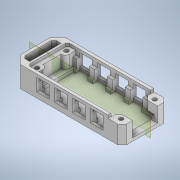
# Autodesk Inventor part: Case_main
Saved by Autodesk Inventor 2020 (Build 240168000, 168)
## iProperties
Created: 2022-03-19
Part Number: Case_main
Material: Типовые
Document SubType Name: Modeling
Designer: NoName
Density: 1 g/cm^3
Appearance: По умолчанию
Author: NoName
Autodesk Inventor part; units mm, degrees
ref_plane "YZ Plane" through (0, 0, 0) normal (1, 0, 0) x (0, 1, 0)
ref_plane "XZ Plane" through (0, 0, 0) normal (0, 1, 0) x (-1, 0, 0)
sketch "Эскиз1" plane through (0, 0, 0) normal (0, 1, 0) x (-1, 0, 0)
  line L0 (0, 0) -> (0, -19)
  line L1 (0, -19) -> (40.8, -19)
  line L2 (40.8, -19) -> (40.8, -15.85)
  arc A0 (42.8, -13.85) -> (40.8, -15.85) centre (42.8, -15.85) ccw
  line L3 (42.8, -15.85) -> (42.8, -13.85) construction
  line L4 (42.8, -15.85) -> (40.8, -15.85) construction
  line L5 (42.8, -13.85) -> (42.8, -5.15)
  line L6 (42.8, -9.5) -> (0, -9.5)
  line L7 (0, 0) -> (40.8, 0)
  line L8 (40.8, 0) -> (40.8, -3.15)
  arc A1 (40.8, -3.15) -> (42.8, -5.15) centre (42.8, -3.15) ccw
  line L9 (42.8, -3.15) -> (42.8, -5.15) construction
  line L10 (42.8, -3.15) -> (40.8, -3.15) construction
  line L11 (46.8, -20.4) -> (0.4, -20.4)
  line L12 (46.8, 1.4) -> (0.4, 1.4)
  line L13 (50.8, -16.4) -> (50.8, -2.6)
  line L14 (45.8, -17) -> (45.8, -2)
  line L15 (49.3, -15.7787) -> (49.3, -3.2213)
  line L16 (5.1, -19) -> (5.1, -17.6)
  line L17 (5.1, -17.6) -> (0, -17.6)
  line L18 (5.1, 0) -> (5.1, -1.4)
  line L19 (5.1, -1.4) -> (0, -1.4)
  line L20 (0.4, -20.4) -> (-1.6, -18.4)
  line L21 (-1.6, -18.4) -> (-1.6, -0.6)
  line L22 (-1.6, -0.6) -> (0.4, 1.4)
  line L23 (46.8, 1.4) -> (50.8, -2.6)
  line L24 (50.8, -16.4) -> (46.8, -20.4)
  line L25 (49.3, -15.7787) -> (48.0787, -17)
  line L26 (48.0787, -17) -> (45.8, -17)
  line L27 (49.3, -3.2213) -> (48.0787, -2)
  line L28 (48.0787, -2) -> (45.8, -2)
  point P0 (5.1, 0)
  point P1 (0, -1.4)
  point P2 (45.8, -9.5)
  point P3 (49.3, -9.5)
  point P4 (50.8, -9.5)
  dimension "d1" = 42.8
  dimension "d3" = 2
  dimension "d4" = 12.7
  dimension "d8" = 19
  dimension "d12" = 3.5
  dimension "d32" = 21.8
  dimension "d34" = 5.1
  dimension "d35" = 16.2
  dimension "d41" = 135
  dimension "d42" = 1.6
  dimension "d43" = 2
  dimension "d65" = 8
  dimension "d66" = 1.5
  dimension "d67" = 15
  dimension "d68" = 1.5
  dimension "d69" = 4
  constraints: 59 end point, 13 symmetric about line, 7 vertical, 6 perpendicular, 5 midpoint, 4 point on circle, 3 horizontal alignment, 2 centre point, 2 point on line, 1 horizontal, 1 parallel, 1 tangent, 1 other
  measures "d1" distance between parallel lines of L0 L5
  measures "d3" distance between parallel lines of L5 L8
  measures "d4" distance of L9.start L3.start
  measures "d8" distance between parallel lines of L7 L1
  measures "d12" distance between parallel lines of L15 L14
  measures "d32" distance between parallel lines of L12 L11
  measures "d34" distance between parallel lines of L0 L16
  measures "d35" distance between parallel lines of L19 L17
  measures "d41" angle of L12 L22
  measures "d42" distance between parallel lines of L0 L21
  measures "d43" horizontal distance of L21.end L12.end
  measures "d65" distance between parallel lines of L5 L13
  measures "d66" distance between parallel lines of L13 L15
  measures "d67" distance between parallel lines of L28 L26
  measures "d68" distance between parallel lines of L24 L25
  measures "d69" distance from line of L5 L11.start
extrude "Выдавливание1" add sketch "Эскиз1" along normal blind 6 contours L7 L18 L19 L0 | L17 L16 L1 L0 | L11 L20 L21 L22 L12 L23 L13 L24
sketch "Эскиз2" plane through (0, 0, 0) normal (0, -1, 0) x (1, 0, 0)
  line L0 (-0.4, -20.4) -> (-46.8, -20.4) projected
  line L1 (-46.8, 1.4) -> (-0.4, 1.4) projected
  line L2 (-50.8, -16.4) -> (-50.8, -2.6) projected
  line L3 (-42.8, -5.15) -> (-42.8, -13.85) projected
  arc A0 (-42.8, -5.15) -> (-40.8, -3.15) centre (-42.8, -3.15) ccw projected
  line L4 (-40.8, 0) -> (-40.8, -3.15) projected
  line L5 (-5.1, 0) -> (-40.8, 0) projected
  line L6 (0, -17.6) -> (0, -1.4) projected
  line L7 (-40.8, -19) -> (-5.1, -19) projected
  line L8 (-40.8, -15.85) -> (-40.8, -19) projected
  arc A1 (-40.8, -15.85) -> (-42.8, -13.85) centre (-42.8, -15.85) ccw projected
  line L9 (-40.8, -15.85) -> (-40.8, -19) projected
  line L10 (-40.8, -19) -> (-5.1, -19) projected
  line L11 (-39.8, -16.8) -> (-1.5, -16.8)
  line L12 (-1.5, -16.8) -> (-1.5, -2.2)
  line L13 (-1.5, -2.2) -> (-39.8, -2.2)
  line L14 (-39.8, -2.2) -> (-39.8, -16.8)
  line L15 (-5.1, -1.4) -> (-5.1, 0) projected
  line L16 (0, -1.4) -> (-5.1, -1.4) projected
  line L17 (-5.1, -17.6) -> (0, -17.6) projected
  line L18 (-5.1, -19) -> (-5.1, -17.6) projected
  line L19 (1.6, -18.4) -> (-0.4, -20.4) projected
  line L20 (1.6, -0.6) -> (1.6, -18.4) projected
  line L21 (-0.4, 1.4) -> (1.6, -0.6) projected
  line L22 (-50.8, -2.6) -> (-46.8, 1.4) projected
  line L23 (-46.8, -20.4) -> (-50.8, -16.4) projected
  line L24 (-49.3, -3.2213) -> (-49.3, -15.7787) projected
  line L25 (-48.0787, -2) -> (-49.3, -3.2213) projected
  line L26 (-45.8, -2) -> (-48.0787, -2) projected
  line L27 (-45.8, -17) -> (-45.8, -2) projected
  line L28 (-48.0787, -17) -> (-45.8, -17) projected
  line L29 (-49.3, -15.7787) -> (-48.0787, -17) projected
  point P0 (0, -18.2)
  point P1 (-42.8, -9.5)
  point P2 (-39.8, -9.5)
  dimension "d17" = 1.5
  dimension "d18" = 3
  dimension "d33" = 14.6
  constraints: 8 end point, 2 midpoint, 2 parallel, 1 horizontal, 1 horizontal alignment, 1 perpendicular, 1 other
  measures "d17" distance between parallel lines of L6 L12
  measures "d18" distance between parallel lines of L3 L14
  measures "d33" distance between parallel lines of L13 L11
extrude "Выдавливание2" add sketch "Эскиз2" along normal blind 1.6 contours L0 L23 L2 L22 L1 L21 L20 L19 | A0 L4 L5 L15 L16 L6 L17 L18 L7 L8 A1 L3
sketch "Эскиз3" plane through (0, -1.6, 0) normal (0, -1, 0) x (1, 0, 0)
  line L0 (-0.4, 1.4) -> (-46.8, 1.4) projected
  line L1 (-50.8, -2.6) -> (-50.8, -16.4) projected
  line L2 (-46.8, -20.4) -> (-0.4, -20.4) projected
  line L3 (-1.5, -2.2) -> (-1.5, -16.8) projected
  line L4 (-1.5, -16.8) -> (-39.8, -16.8) projected
  line L5 (-39.8, -16.8) -> (-39.8, -2.2) projected
  line L6 (-39.8, -2.2) -> (-1.5, -2.2) projected
  line L7 (-0.4, -20.4) -> (1.6, -18.4) projected
  line L8 (1.6, -18.4) -> (1.6, -0.6) projected
  line L9 (1.6, -0.6) -> (-0.4, 1.4) projected
  line L10 (-46.8, 1.4) -> (-50.8, -2.6) projected
  line L11 (-50.8, -16.4) -> (-46.8, -20.4) projected
  line L12 (-49.3, -15.7787) -> (-49.3, -3.2213) projected
  line L13 (-49.3, -3.2213) -> (-48.0787, -2) projected
  line L14 (-48.0787, -2) -> (-45.8, -2) projected
  line L15 (-45.8, -2) -> (-45.8, -17) projected
  line L16 (-45.8, -17) -> (-48.0787, -17) projected
  line L17 (-48.0787, -17) -> (-49.3, -15.7787) projected
  point P0 (0, 0)
extrude "Выдавливание3" add sketch "Эскиз3" along normal blind 1 contours L9 L8 L7 L2 L11 L1 L10 L0 | L3 L4 L5 L6
sketch "Эскиз5" plane through (-46.8, 6, 1.4) normal (0, 0, 1) x (1, 0, 0)
  line L0 (7.8, 0) -> (13.8, 0)
  line L1 (13.8, 0) -> (13.8, -6)
  line L2 (13.8, -6) -> (7.8, -6)
  line L3 (7.8, -6) -> (7.8, 0)
  line L4 (0, 0) -> (46.4, 0) projected
  line L5 (4, -6) -> (4, 0) projected
  point P0 (46.8, -6)
  point P1 (46.5, 0)
  dimension "d27" = 6
  dimension "d28" = 6
  dimension "d29" = 3.8
  constraints: 8 end point, 2 parallel, 1 horizontal, 1 perpendicular, 1 point on line
  measures "d27" distance between parallel lines of L3 L1
  measures "d28" distance between parallel lines of L0 L2
  measures "d29" distance between parallel lines of L5 L3
extrude "Выдавливание5" cut sketch "Эскиз5" against normal through all
pattern_linear "Прямоуг.массив1" count 4 spacing 8.5 along (1, 0, 0) of "Выдавливание5"
sketch "Эскиз6" plane through (0, 0, 0) normal (0, 1, 0) x (1, 0, 0)
  line L0 (-5.1, 0) -> (-40.8, 0) projected
  line L1 (-16, 0) -> (-13.5, 0)
  line L2 (-13.5, 0) -> (-13.5, 1.4)
  line L3 (-13.5, 1.4) -> (-16, 1.4)
  line L4 (-16, 1.4) -> (-16, 0)
  line L5 (-24.5, 0) -> (-22, 0)
  line L6 (-22, 0) -> (-22, 1.4)
  line L7 (-22, 1.4) -> (-24.5, 1.4)
  line L8 (-24.5, 1.4) -> (-24.5, 0)
  line L9 (-33, 0) -> (-30.5, 0)
  line L10 (-30.5, 0) -> (-30.5, 1.4)
  line L11 (-30.5, 1.4) -> (-33, 1.4)
  line L12 (-33, 1.4) -> (-33, 0)
  line L13 (-39, 0) -> (-40.8, 0)
  line L14 (-40.8, 0) -> (-40.8, 1.4)
  line L15 (-40.8, 1.4) -> (-39, 1.4)
  line L16 (-39, 1.4) -> (-39, 0)
  line L17 (-5.1, 0) -> (-7.5, 0) projected
  line L18 (-5.1, 0) -> (-7.5, 0) projected
  line L19 (-39, 0) -> (-40.8, 0) projected
  line L20 (0, 1.4) -> (-5.1, 1.4) projected
  line L21 (-7.5, 0) -> (-5.1, 0)
  line L22 (-5.1, 0) -> (-5.1, 1.4)
  line L23 (-5.1, 1.4) -> (-7.5, 1.4)
  line L24 (-7.5, 1.4) -> (-7.5, 0)
  line L25 (-42.8, 5.15) -> (-42.8, 13.85) projected
  line L26 (-42.8, 9.5) -> (-1.5, 9.5)
  line L27 (-5.1, 19) -> (-40.8, 19)
  line L28 (-16, 19) -> (-13.5, 19)
  line L29 (-13.5, 19) -> (-13.5, 17.6)
  line L30 (-13.5, 17.6) -> (-16, 17.6)
  line L31 (-16, 17.6) -> (-16, 19)
  line L32 (-24.5, 19) -> (-22, 19)
  line L33 (-22, 19) -> (-22, 17.6)
  line L34 (-22, 17.6) -> (-24.5, 17.6)
  line L35 (-24.5, 17.6) -> (-24.5, 19)
  line L36 (-33, 19) -> (-30.5, 19)
  line L37 (-30.5, 19) -> (-30.5, 17.6)
  line L38 (-30.5, 17.6) -> (-33, 17.6)
  line L39 (-33, 17.6) -> (-33, 19)
  line L40 (-39, 19) -> (-40.8, 19)
  line L41 (-40.8, 19) -> (-40.8, 17.6)
  line L42 (-40.8, 17.6) -> (-39, 17.6)
  line L43 (-39, 17.6) -> (-39, 19)
  line L44 (-5.1, 19) -> (-7.5, 19)
  line L45 (-5.1, 19) -> (-40.8, 19)
  line L46 (-39, 19) -> (-40.8, 19)
  line L47 (-39, 19) -> (-33, 19)
  line L48 (-30.5, 19) -> (-33, 19)
  line L49 (-30.5, 19) -> (-24.5, 19)
  line L50 (-22, 19) -> (-24.5, 19)
  line L51 (-22, 19) -> (-16, 19)
  line L52 (-13.5, 19) -> (-16, 19)
  line L53 (0, 17.6) -> (-5.1, 17.6)
  line L54 (-7.5, 19) -> (-5.1, 19)
  line L55 (-5.1, 19) -> (-5.1, 17.6)
  line L56 (-5.1, 17.6) -> (-7.5, 17.6)
  line L57 (-7.5, 17.6) -> (-7.5, 19)
  line L58 (-1.5, 2.2) -> (-1.5, 16.8) projected
  line L59 (-30.5, 0) -> (-33, 0) projected
  line L60 (-22, 0) -> (-24.5, 0) projected
  line L61 (-13.5, 0) -> (-16, 0) projected
  line L62 (-13.5, 0) -> (-16, 0) projected
  line L63 (-39, 0) -> (-40.8, 0) projected
  line L64 (-22, 0) -> (-24.5, 0) projected
  line L65 (-30.5, 0) -> (-33, 0) projected
  point P0 (0, 0)
  point P1 (0, 19)
  point P2 (-5.1, 19)
  point P3 (-7.1397, 18.6)
  point P4 (-22, 19)
  point P5 (-30.5, 19)
  point P6 (-7.5, 0)
  point P7 (-13.5, 0)
  point P8 (-22, 0)
  point P9 (-30.5, 0)
  point P10 (-7.5, 19)
  constraints: 104 end point, 29 symmetric about line, 11 point on line, 10 parallel, 6 horizontal, 5 perpendicular, 4 horizontal alignment, 2 midpoint
extrude "Выдавливание6" add sketch "Эскиз6" along normal blind 4
sketch "Эскиз7" plane through (1.6, 6, -0.6) normal (1, 0, 0) x (0, 0, -1)
  line L0 (16.4, 0) -> (1.4, 0) projected
  line L1 (14.9, 0) -> (2.9, 0)
  line L2 (2.9, 0) -> (2.9, -7.1)
  line L3 (2.9, -7.1) -> (14.9, -7.1)
  line L4 (14.9, -7.1) -> (14.9, 0)
  point P0 (-0.6, -6)
  point P1 (16.5, 0)
  point P2 (-0.5, 0)
  point P3 (8.9, 0)
  point P4 (2.9, 0)
  dimension "d44" = 12
  dimension "d45" = 7.1
  constraints: 8 end point, 2 midpoint, 2 parallel, 1 horizontal, 1 perpendicular, 1 point on line
  measures "d44" distance between parallel lines of L4 L2
  measures "d45" distance between parallel lines of L3 L0
extrude "Выдавливание7" cut sketch "Эскиз7" against normal up to next
ref_plane "РабПлоскость1" through (0, 1.8, 0) normal (0, 1, 0) x (1, 0, 0)
sketch "Эскиз8" plane through (0, 1.8, 0) normal (0, 1, 0) x (1, 0, 0)
  line L0 (0, 17.6) -> (0, 15.5) projected
  line L1 (0, 17.6) -> (-5.1, 17.6)
  line L2 (0, 15.5) -> (0, 17.6)
  line L3 (-42.8, 5.15) -> (-42.8, 13.85) projected
  line L4 (-42.8, 9.5) -> (1.6, 9.5)
  line L5 (-5.1, 17.6) -> (-3, 15.5)
  line L6 (-3, 15.5) -> (0, 15.5)
  line L7 (0, 17.6) -> (-7.5, 17.6) projected
  line L8 (0, 1.4) -> (0, 3.5)
  line L9 (0, 1.4) -> (-5.1, 1.4)
  line L10 (0, 3.5) -> (0, 1.4)
  line L11 (-5.1, 1.4) -> (-3, 3.5)
  line L12 (-3, 3.5) -> (0, 3.5)
  line L13 (1.6, 15.5) -> (1.6, 3.5) projected
  point P0 (0, 0)
  dimension "d49" = 45
  constraints: 20 end point, 5 symmetric about line, 2 midpoint, 2 point on line, 1 horizontal, 1 parallel
  measures "d49" angle of L1 L5
extrude "Выдавливание8" add sketch "Эскиз8" along normal up to surface (4.2 mm away)
sketch "Эскиз10" plane through (0, 6, 0) normal (0, 1, 0) x (1, 0, 0)
  line L0 (-42.8, 5.15) -> (-42.8, 13.85) projected
  line L1 (-42.8, 9.5) -> (-1.5, 9.5)
  line L2 (-1.5, 2.2) -> (-1.5, 16.8) projected
  line L3 (-45.8, 17) -> (-45.8, 2) projected
  line L4 (1.6, 15.5) -> (1.6, 18.4) projected
  point P0 (0, 0)
  point P1 (-42.8, 16.5)
  point P2 (-42.8, 2.5)
  point P3 (-1.8, 17.5)
  point P4 (-1.8, 1.5)
  point P5 (-44.8, 17.7)
  point P6 (-44.8, 0.7)
  point P7 (-45.8, 2)
  dimension "d59" = 16
  dimension "d60" = 14
  dimension "d62" = 3.4
  dimension "d76" = 41
  constraints: 2 end point, 2 midpoint, 2 symmetric about line, 1 other
  measures "d59" distance of point (-1.8, 1.5) point (-1.8, 17.5)
  measures "d60" distance of point (-42.8, 2.5) point (-42.8, 16.5)
  measures "d62" distance from line of L4 point (-1.8, 17.5)
  measures "d76" horizontal distance of point (-42.8, 16.5) point (-1.8, 17.5)
hole "Отверстие1" at (-42.8, 6, -16.5) at (-42.8, 6, -2.5) at (-1.8, 6, -17.5) at (-1.8, 6, -1.5) direction (0, -1, 0) diameter 2 depth 6
sketch "Эскиз13" plane through (0, 6, 0) normal (0, 1, 0) x (1, 0, 0)
  circle A0 centre (-42.8, 16.5) radius 1 projected
  circle A1 centre (-42.8, 2.5) radius 1 projected
  line L0 (-48.0787, 2) -> (-49.3, 3.2213) projected
  line L1 (-49.3, 3.2213) -> (-49.3, 15.7787) projected
  line L2 (-49.3, 15.7787) -> (-48.0787, 17) projected
  line L3 (-48.0787, 17) -> (-45.8, 17) projected
  line L4 (-45.8, 17) -> (-45.8, 2) projected
  line L5 (-45.8, 2) -> (-48.0787, 2) projected
  line L6 (-50.8, 2.6) -> (-46.8, -1.4) projected
  line L7 (-46.8, -1.4) -> (-39, -1.4) projected
  line L8 (-39, -1.4) -> (-39, 0) projected
  line L9 (-39, 0) -> (-40.8, 0) projected
  line L10 (-40.8, 0) -> (-40.8, 3.15) projected
  arc A2 (-40.8, 3.15) -> (-42.8, 5.15) centre (-42.8, 3.15) ccw projected
  line L11 (-42.8, 5.15) -> (-42.8, 13.85) projected
  arc A3 (-42.8, 13.85) -> (-40.8, 15.85) centre (-42.8, 15.85) ccw projected
  line L12 (-40.8, 15.85) -> (-40.8, 19) projected
  line L13 (-40.8, 19) -> (-39, 19) projected
  line L14 (-39, 19) -> (-39, 20.4) projected
  line L15 (-39, 20.4) -> (-46.8, 20.4) projected
  line L16 (-46.8, 20.4) -> (-50.8, 16.4) projected
  line L17 (-50.8, 16.4) -> (-50.8, 2.6) projected
  line L18 (-40.8, 19) -> (-39, 19) projected
  line L19 (-5.1, 19) -> (-5.1, 17.6) projected
  line L20 (-39, 0) -> (-40.8, 0) projected
  line L21 (-39, -1.4) -> (-39, 0) projected
  line L22 (-40.8, 0) -> (-40.8, 1.4) projected
  line L23 (-40.8, 19) -> (-43.8, 19)
  line L24 (-43.8, 19) -> (-44.8, 18)
  line L25 (-44.8, 18) -> (-44.8, 1)
  line L26 (-44.8, 1) -> (-43.8, 0)
  line L27 (-43.8, 0) -> (-40.8, 0)
  line L28 (-42.8, 5.15) -> (-42.8, 13.85) projected
  line L29 (-42.8, 9.5) -> (-1.5, 9.5)
  line L30 (-1.5, 2.2) -> (-1.5, 16.8) projected
  line L31 (-40.8, 19) -> (-39, 19) projected
  line L32 (-5.1, 19) -> (-39, 19)
  line L33 (-5.1, 19) -> (-5.1, 20.4)
  line L34 (-46.8, 20.4) -> (-0.4, 20.4) projected
  line L35 (-39, 20.4) -> (-46.8, 20.4) projected
  line L36 (-5.1, 20.4) -> (-39, 20.4)
  line L37 (-5.1, 0) -> (-39, 0)
  line L38 (-39, 1.4) -> (-39, -1.4) projected
  line L39 (-5.1, 0) -> (-5.1, -1.4)
  line L40 (-0.4, -1.4) -> (-46.8, -1.4) projected
  line L41 (-5.1, -1.4) -> (-39, -1.4)
  point P0 (0, 0)
  dimension "d71" = 1
  dimension "d72" = 1
  constraints: 24 end point, 5 perpendicular, 2 horizontal, 2 midpoint, 2 point on line, 2 vertical, 1 collinear, 1 parallel, 1 other
  measures "d71" distance between parallel lines of L4 L25
  measures "d72" horizontal distance of L23.end L24.end
extrude "Выдавливание9" add sketch "Эскиз13" along normal blind 1.4 contours L17 L16 L15 L14 L13 L23 L24 L25 L26 L27 L9 L8 L7 L6 | L8 L37 L39 L40 | L34 L33 L32 L14
sketch "Эскиз16" plane through (1.6, -1.1, -3.5) normal (0, 0, -1) x (-1, 0, 0)
  line L0 (4.4, 2.9) -> (2.4, 2.9) projected
  line L1 (4.5, 2.9) -> (6.7, 5.1)
  line L2 (6.7, 5.1) -> (6.7, 2.9) projected
  line L3 (6.7, 5.1) -> (6.7, 2.9)
  line L4 (4.5, 2.9) -> (6.7, 2.9)
  point P0 (1.6, 1.1)
  point P1 (2.405, 2.9)
  point P2 (4.395, 2.9)
  point P3 (4.4, 2.9)
  constraints: 6 end point, 2 perpendicular, 1 collinear, 1 point on line
extrude "Выдавливание11" cut sketch "Эскиз16" against normal up to surface (2.1 mm away)
sketch "Эскиз17" plane through (-1.5, 0, -2.2) normal (0, 0, -1) x (-1, 0, 0)
  line L0 (3.6, 4) -> (6, 4) projected
  line L1 (6, 4) -> (6, 6) projected
  line L2 (6, 6) -> (12, 6) projected
  line L3 (12, 6) -> (12, 4) projected
  line L4 (12, 4) -> (14.5, 4) projected
  line L5 (14.5, 4) -> (14.5, 6) projected
  line L6 (14.5, 6) -> (20.5, 6) projected
  line L7 (20.5, 6) -> (20.5, 4) projected
  line L8 (20.5, 4) -> (23, 4) projected
  line L9 (23, 4) -> (23, 6) projected
  line L10 (23, 6) -> (29, 6) projected
  line L11 (29, 6) -> (29, 4) projected
  line L12 (29, 4) -> (31.5, 4) projected
  line L13 (31.5, 4) -> (31.5, 6) projected
  line L14 (31.5, 6) -> (37.5, 6) projected
  line L15 (37.5, 6) -> (37.5, 4) projected
  line L16 (37.5, 4) -> (39.3, 4) projected
  line L17 (39.3, 4) -> (39.3, 6) projected
  line L18 (42.3, 6) -> (39.3, 6) projected
  line L19 (42.3, 6) -> (42.3, 7.4) projected
  line L20 (3.6, 7.4) -> (42.3, 7.4) projected
  line L21 (3.6, 6) -> (3.6, 7.4) projected
  line L22 (3.6, 4) -> (3.6, 6) projected
  line L23 (38.3, 0) -> (0, 0) projected
  line L24 (0, 0) -> (0, -1.6) projected
  line L25 (38.3, -1.6) -> (0, -1.6) projected
  line L26 (38.3, 0) -> (38.3, -1.6) projected
  line L27 (38.3, 0) -> (0, 0) projected
  line L28 (38.3, -1.6) -> (0, -1.6) projected
  line L29 (6, 0) -> (12, 0)
  line L30 (12, 0) -> (12, -1.6)
  line L31 (12, -1.6) -> (6, -1.6)
  line L32 (6, -1.6) -> (6, 0)
  line L33 (14.5, 0) -> (20.5, 0)
  line L34 (20.5, 0) -> (20.5, -1.6)
  line L35 (20.5, -1.6) -> (14.5, -1.6)
  line L36 (14.5, -1.6) -> (14.5, 0)
  line L37 (23, 6) -> (23, 0) projected
  line L38 (23, 0) -> (29, 0)
  line L39 (29, 0) -> (29, -1.6)
  line L40 (29, -1.6) -> (23, -1.6)
  line L41 (23, -1.6) -> (23, 0)
  line L42 (31.5, 6) -> (31.5, 0) projected
  line L43 (31.5, 0) -> (37.5, 0)
  line L44 (37.5, 0) -> (37.5, -1.6)
  line L45 (37.5, -1.6) -> (31.5, -1.6)
  line L46 (31.5, -1.6) -> (31.5, 0)
  point P0 (-1.5, 0)
  point P1 (37.5, -1.6)
  point P2 (14.5, -1.6)
  point P3 (6, -1.6)
  constraints: 32 end point, 8 parallel, 7 point on line, 4 horizontal, 4 perpendicular
extrude "Выдавливание12" cut sketch "Эскиз17" against normal up to surface (2.2 mm away) contours L23 L39 L25 L41 | L34 L25 L36 L23 | L23 L44 L25 L46 | L30 L25 L32 L23
ref_plane "РабПлоскость2" through (1.6, -1.1, -9.5) normal (0, 0, -1) x (-1, 0, 0)
mirror "Зеркальное отражение1" about plane through (1.6, -1.1, -9.5) normal (0, 0, -1) of "Выдавливание12", "Выдавливание11"
